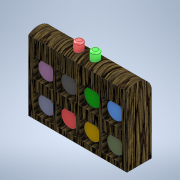
# Autodesk Inventor part: TreasureChestFinal
Saved by Autodesk Inventor 2021 (Build 250183000, 183)
## iProperties
Created: 2021-03-02
Part Number: TreasureChestFinal
Material: Generic
Document SubType Name: Modeling
Designer: con_c_000
Density: 1 g/cm^3
Appearance: Default
Author: con_c_000
Autodesk Inventor part; units mm, degrees
ref_plane "YZ Plane" through (0, 0, 0) normal (1, 0, 0) x (0, 1, 0)
ref_plane "XZ Plane" through (0, 0, 0) normal (0, 1, 0) x (-1, 0, 0)
ref_plane "XY Plane" through (0, 0, 0) normal (0, 0, 1) x (1, 0, 0)
sketch "Sketch1" plane through (0, 0, 0) normal (0, 1, 0) x (-1, 0, 0)
  line L0 (923.5659, 4.2179) -> (-600.4341, 4.2179)
  line L1 (-600.4341, 4.2179) -> (-600.4341, -300.5821)
  line L2 (-600.4341, -300.5821) -> (923.5659, -300.5821)
  line L3 (923.5659, -300.5821) -> (923.5659, 4.2179)
  point P0 (0, 0)
  dimension "d0" = 1524
  dimension "d1" = 304.8
  constraints: 8 end point, 2 parallel, 1 horizontal, 1 perpendicular
  measures "d0" distance of L2.end L1.end
  measures "d1" distance of L1.end L0.end
extrude "Extrusion1" add sketch "Sketch1" along normal blind 914.4
sketch "Sketch2" plane through (-923.5659, 0, 4.2179) normal (0, 0, 1) x (1, 0, 0)
  circle A0 centre (228.6, 228.6) radius 127
  circle A1 centre (584.2, 228.6) radius 127
  circle A2 centre (939.8, 228.6) radius 127
  circle A3 centre (1295.4, 228.6) radius 127
  circle A4 centre (1295.4, 685.8) radius 127
  circle A5 centre (939.8, 685.8) radius 127
  circle A6 centre (584.2, 685.8) radius 127
  circle A7 centre (228.6, 685.8) radius 127
  line L0 (1524, 0) -> (1524, 914.4) projected
  line L1 (0, 0) -> (0, 914.4) projected
  line L2 (0, 914.4) -> (1524, 914.4) projected
  point P0 (923.5659, 0)
  dimension "d11" = 254
  dimension "d19" = 355.6
  dimension "d20" = 355.6
  dimension "d21" = 228.6
  dimension "d22" = 457.2
  dimension "d23" = 355.6
  dimension "d24" = 228.6
  constraints: 8 centre point, 7 equal radius, 6 horizontal alignment, 4 vertical alignment
  measures "d11" diameter of A7
  measures "d19" distance of A6.centre A5.centre
  measures "d20" distance of A4.centre A5.centre
  measures "d21" distance from line of L2 A7.centre
  measures "d22" distance of A0.centre A7.centre
  measures "d23" distance of A6.centre A7.centre
  measures "d24" distance from line of L1 A7.centre
extrude "Extrusion2" add sketch "Sketch2" along normal blind 25.4
sketch "Sketch3" plane through (-923.5659, 0, 4.2179) normal (0, 0, 1) x (1, 0, 0)
  line L0 (0, 914.4) -> (1524, 914.4) projected
  line L1 (0, 914.4) -> (1524, 914.4)
  line L2 (1524, 914.4) -> (1524, 0)
  line L3 (1524, 0) -> (0, 0)
  line L4 (0, 0) -> (0, 914.4)
  line L5 (76.2, 838.2) -> (381, 838.2)
  line L6 (381, 838.2) -> (381, 533.4)
  line L7 (381, 533.4) -> (76.2, 533.4)
  line L8 (76.2, 533.4) -> (76.2, 838.2)
  line L9 (431.8, 533.4) -> (736.6, 533.4)
  line L10 (736.6, 533.4) -> (736.6, 838.2)
  line L11 (736.6, 838.2) -> (431.8, 838.2)
  line L12 (431.8, 838.2) -> (431.8, 533.4)
  line L13 (787.4, 838.2) -> (1092.2, 838.2)
  line L14 (1092.2, 838.2) -> (1092.2, 533.4)
  line L15 (1092.2, 533.4) -> (787.4, 533.4)
  line L16 (787.4, 533.4) -> (787.4, 838.2)
  line L17 (1143, 533.4) -> (1447.8, 533.4)
  line L18 (1447.8, 533.4) -> (1447.8, 838.2)
  line L19 (1447.8, 838.2) -> (1143, 838.2)
  line L20 (1143, 838.2) -> (1143, 533.4)
  line L21 (76.2, 381) -> (381, 381)
  line L22 (381, 381) -> (381, 76.2)
  line L23 (381, 76.2) -> (76.2, 76.2)
  line L24 (76.2, 76.2) -> (76.2, 381)
  line L25 (431.8, 76.2) -> (736.6, 76.2)
  line L26 (736.6, 76.2) -> (736.6, 381)
  line L27 (736.6, 381) -> (431.8, 381)
  line L28 (431.8, 381) -> (431.8, 76.2)
  line L29 (787.4, 381) -> (1092.2, 381)
  line L30 (1092.2, 381) -> (1092.2, 76.2)
  line L31 (1092.2, 76.2) -> (787.4, 76.2)
  line L32 (787.4, 76.2) -> (787.4, 381)
  line L33 (1143, 76.2) -> (1447.8, 76.2)
  line L34 (1447.8, 76.2) -> (1447.8, 381)
  line L35 (1447.8, 381) -> (1143, 381)
  line L36 (1143, 381) -> (1143, 76.2)
  line L37 (0, 0) -> (1524, 0) projected
  point P0 (923.5659, 0)
  dimension "d25" = 304.8
  dimension "d26" = 304.8
  dimension "d27" = 76.2
  dimension "d28" = 50.8
  dimension "d29" = 76.2
  dimension "d30" = 50.8
  dimension "d31" = 50.8
  dimension "d32" = 0
  dimension "d33" = 0
  dimension "d34" = 0
  dimension "d35" = 304.8
  dimension "d36" = 152.4
  dimension "d37" = 0
  dimension "d52" = 0
  constraints: 72 end point, 17 parallel, 13 point on line, 10 horizontal, 9 perpendicular, 5 equal length, 1 collinear
  measures "d25" distance of L5.start L5.end
  measures "d26" distance of L7.end L5.start
  measures "d27" distance between parallel lines of L0 L5
  measures "d28" distance between parallel lines of L6 L12
  measures "d29" distance between parallel lines of L4 L8
  measures "d30" distance between parallel lines of L16 L10
  measures "d31" distance between parallel lines of L20 L14
  measures "d32" distance between parallel lines of L13 L19
  measures "d33" distance between parallel lines of L34 L18
  measures "d34" distance between parallel lines of L27 L21
  measures "d35" distance of L23.end L21.start
  measures "d36" distance between parallel lines of L7 L21
  measures "d37" distance between parallel lines of L25 L31
  measures "d52" distance between parallel lines of L24 L8
extrude "Extrusion3" add sketch "Sketch3" along normal blind 76.2
sketch "Sketch5" plane through (0, 914.4, 0) normal (0, 1, 0) x (1, 0, 0)
  line L0 (600.4341, 300.5821) -> (600.4341, -80.4179) projected
  line L1 (600.4341, 300.5821) -> (-923.5659, 300.5821) projected
  line L2 (-923.5659, 300.5821) -> (-923.5659, -80.4179) projected
  line L3 (600.4341, -80.4179) -> (-923.5659, -80.4179) projected
  point P0 (0, 0)
extrude "Extrusion4" add sketch "Sketch5" along normal blind 254
sketch "Sketch6" plane through (-923.5659, 0, -300.5821) normal (-1, 0, 0) x (0, 0, 1)
  line L0 (381, 0) -> (381, 1168.4) projected
  line L1 (0, 0) -> (0, 1168.4) projected
  arc A0 (381, 1083.587) -> (0, 944.9143) centre (234.5045, 893.3493) ccw
  line L2 (381, 1083.587) -> (0, 944.9143) construction
  line L3 (381, 1083.587) -> (786.4517, 1083.587) construction
  line L4 (0, 944.9143) -> (381, 944.9143)
  line L5 (381, 944.9143) -> (381, 1168.4)
  line L6 (381, 1168.4) -> (0, 1168.4)
  line L7 (0, 1168.4) -> (0, 944.9143)
  point P0 (300.5821, 0)
  point P1 (0, 1168.4)
  point P2 (0, 971.0107)
  dimension "d42" = 160
  constraints: 12 end point, 2 horizontal, 2 parallel, 2 point on circle, 2 point on line, 1 centre point, 1 equal length, 1 perpendicular
  measures "d42" angle of L2 L3
extrude "Extrusion5" cut sketch "Sketch6" against normal through all contours A0 L1 L6 L0
ref_plane "Work Plane1" through (-923.5659, 1133.4562, -66.0776) normal (0, -1, 0) x (1, 0, 0)
sketch "Sketch7" plane through (-923.5659, 1133.4562, -66.0776) normal (0, -1, 0) x (1, 0, 0)
  circle A0 centre (635, 0.1041) radius 63.5
  circle A1 centre (889, 0.1041) radius 63.5
  line L0 (1524, -234.5045) -> (1524, 146.4955) projected
  line L1 (0, 146.4955) -> (0, -234.5045) projected
  point P0 (923.5659, 66.0776)
  dimension "d45" = 127
  dimension "d46" = 127
  dimension "d47" = 635
  dimension "d48" = 635
  constraints: 2 centre point
  measures "d45" diameter of A0
  measures "d46" diameter of A1
  measures "d47" distance from line of L0 A1.centre
  measures "d48" distance from line of L1 A0.centre
extrude "Extrusion6" add sketch "Sketch7" along normal mid plane 254 from surface at 0
fillet "Fillet1" radius 25.4 2 edges at (-352.0659, 1260.4562, -65.9734) (-98.0659, 1260.4562, -65.9734)
equation "\"d19\" = d14"
equation "\"d20\" = d14"
equation "\"d22\" = 2 * d21"
equation "\"d23\" = d14"
equation "\"d30\" = d28"
equation "\"d31\" = d28"
equation "\"d14\" = 355.6"
body "Solid1"
